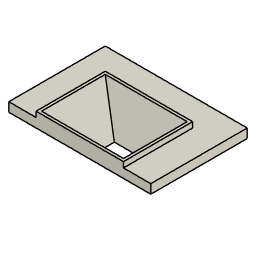
smarties_hopper (Autodesk Fusion 360 design; units mm, degrees)
part number: 2025-05-19-10-29-37-314
Autodesk Fusion 360 part; units mm, degrees
sketch "Bottom opening" plane through (0, 0, 0) normal (0, 0, 1) x (1, 0, 0)
  line L0 (0, 0) -> (25, 0)
  line L1 (25, 0) -> (25, 25)
  line L2 (25, 25) -> (0, 25)
  line L3 (0, 25) -> (0, 0)
  line L4 (-4, 29) -> (29, 29)
  line L5 (29, 29) -> (29, -4)
  line L6 (29, -4) -> (-4, -4)
  line L7 (-4, -4) -> (-4, 29)
  dimension "d3" = 25
  dimension "d4" = 25
  dimension "d5" = 4
  dimension "d6" = 4
  dimension "d7" = 4
  dimension "d8" = 4
  constraint horizontal L0
  constraint vertical L1
  constraint horizontal L2
  constraint vertical L3
  constraint coincident L0.start L3.end
  constraint horizontal L4
  constraint vertical L5
  constraint horizontal L6
  constraint vertical L7
  measures "d3" distance of L0.start L0.end
  measures "d4" distance of L0.end L1.end
  measures "d5" distance of L2 L4
  measures "d6" distance of L0 L6
  measures "d7" distance of L1 L5
  measures "d8" distance of L3 L7
ref_plane "WorkPlane1" through (0, 0, 37) normal (0, 0, 1) x (1, 0, 0)
sketch "Top opening" plane through (0, 0, 37) normal (0, 0, 1) x (1, 0, 0)
  line L0 (25, 25) -> (0, 25)
  line L1 (25, 0) -> (25, 25)
  line L2 (0, 0) -> (25, 0)
  line L3 (0, 25) -> (0, 0)
  line L4 (-4, 29) -> (29, 29)
  line L5 (29, -4) -> (-4, -4)
  line L6 (29, 29) -> (29, -4)
  line L7 (-4, -4) -> (-4, 29)
  line L8 (-32.5, 47.5) -> (57.5, 47.5)
  line L9 (57.5, 47.5) -> (57.5, -22.5)
  line L10 (57.5, -22.5) -> (-32.5, -22.5)
  line L11 (-32.5, -22.5) -> (-32.5, 47.5)
  line L12 (-35.5, 50.5) -> (60.5, 50.5)
  line L13 (60.5, 50.5) -> (60.5, -25.5)
  line L14 (60.5, -25.5) -> (-35.5, -25.5)
  line L15 (-35.5, -25.5) -> (-35.5, 50.5)
  line L16 (-36.5, 51.5) -> (61.5, 51.5)
  line L17 (61.5, 51.5) -> (61.5, -26.5)
  line L18 (61.5, -26.5) -> (-36.5, -26.5)
  line L19 (-36.5, -26.5) -> (-36.5, 51.5)
  dimension "d14" = 3
  dimension "d15" = 4
  dimension "d16" = 3
  dimension "d17" = 4
  dimension "d18" = 90
  dimension "d19" = 70
  dimension "d20" = 3
  dimension "d21" = 4
  dimension "d22" = 3
  dimension "d23" = 4
  dimension "d24" = 28.5
  dimension "d25" = 28.5
  dimension "d26" = 18.5
  dimension "d27" = 18.5
  constraint horizontal L8
  constraint vertical L9
  constraint horizontal L10
  constraint vertical L11
  constraint horizontal L12
  constraint vertical L13
  constraint horizontal L14
  constraint vertical L15
  constraint horizontal L16
  constraint vertical L17
  constraint horizontal L18
  constraint vertical L19
  measures "d14" distance of L9 L13
  measures "d15" distance of L9 L17
  measures "d16" distance of L11 L15
  measures "d17" distance of L11 L19
  measures "d18" distance of L8.start L8.end
  measures "d19" distance of L8.end L9.end
  measures "d20" distance of L8 L12
  measures "d21" distance of L8 L16
  measures "d22" distance of L10 L14
  measures "d23" distance of L10 L18
  measures "d24" distance of L7 L11
  measures "d25" distance of L6 L9
  measures "d26" distance of L4 L8
  measures "d27" distance of L5 L10
loft "Loft1" add profiles "Top opening", "Bottom opening" section 1 contours L8 L9 L10 L11 | L12 L13 L14 L15 | L16 L17 L18 L19 section 2 contours L0 L1 L2 L3 | L4 L5 L6 L7
extrude "Extrude1" cut sketch "Top opening" against normal blind 6 contours L16 L17 L18 L19
sketch "Support lip" plane through (60.5, 0, 0) normal (1, 0, 0) x (0, 1, 0)
  line L0 (-25.5, 35.8615) -> (50.5, 35.8615)
  line L1 (50.5, 35.8615) -> (50.5, 37)
  line L2 (50.5, 37) -> (-25.5, 37)
  line L3 (-25.5, 37) -> (-25.5, 35.8615)
  line L4 (-25.5, 31) -> (80.5, 31)
  line L5 (80.5, 31) -> (80.5, 21)
  line L6 (80.5, 21) -> (-25.5, 21)
  line L7 (-25.5, 21) -> (-25.5, 31)
  dimension "d31" = 6
  dimension "d34" = 10
  dimension "d35" = 30
  constraint horizontal L4
  constraint vertical L5
  constraint horizontal L6
  constraint vertical L7
  constraint collinear L3 L7
  measures "d31" distance of L2 L4
  measures "d34" distance of L4.start L6.end
  measures "d35" horizontal distance of L1.end L4.end
extrude "Extrude2" add sketch "Support lip" along normal blind 30 and the other way blind 126 contours L4 L5 L6 L7
loft "Loft2" cut profiles "Top opening", "Bottom opening" section 1 contours L8 L9 L10 L11 section 2 contours L0 L1 L2 L3
extrude "Extrude3" add 1 faces at (-2.5, 49.5, 37) along direction (0, 0, -1) blind 6
equation "bottom_outlet_size = 25 mm" comment "The side lengths of the bottom opening of the Smartie Hopper."
equation "hopper_wall_thickness = 4 mm" comment "The thickness of the hopper walls used for the \"loft\" function."
equation "d3 = bottom_outlet_size"
equation "d4 = bottom_outlet_size"
equation "d5 = hopper_wall_thickness"
equation "d6 = hopper_wall_thickness"
equation "d7 = hopper_wall_thickness"
equation "d8 = hopper_wall_thickness"
equation "hopper_height = 37 mm" comment "Distance between the top and bottom openings of the Smartie Hopper."
equation "d10 = hopper_height"
equation "acrylic_thickness = 3 mm" comment "Thickness of the clear acrylic panels used for the Unsorted Smarties Holder."
equation "top_outlet_width = 90 mm" comment "The width of the top opening of the Smartie Hopper."
equation "top_outlet_depth = 70 mm" comment "The depth of the top opening of the Smartie Hopper."
equation "d14 = acrylic_thickness"
equation "d15 = hopper_wall_thickness"
equation "d16 = acrylic_thickness"
equation "d17 = hopper_wall_thickness"
equation "d18 = top_outlet_width"
equation "d19 = top_outlet_depth"
equation "d20 = acrylic_thickness"
equation "d21 = hopper_wall_thickness"
equation "d22 = acrylic_thickness"
equation "d23 = hopper_wall_thickness"
equation "d24 = ( top_outlet_width - ( bottom_outlet_size + 2 * hopper_wall_thickness ) ) / 2"
equation "d26 = ( top_outlet_depth - ( bottom_outlet_size + 2 * hopper_wall_thickness ) ) / 2"
equation "MDF_thickness = 6 mm" comment "Thickness of the MDF panels used for the construction of the mini arcade game enclosure."
equation "d29 = -MDF_thickness"
equation "d31 = MDF_thickness"
equation "support_lip_width = 30 mm" comment "The depth that the suport lip should extend beneath the Colour Detection Mechanism Top Panel."
equation "support_lip_thickness = 10 mm" comment "The thickness of the support lip."
equation "d34 = support_lip_thickness"
equation "d35 = support_lip_width"
equation "d36 = support_lip_width"
equation "d38 = ( top_outlet_width + 2 * acrylic_thickness ) + support_lip_width"
equation "d40 = -MDF_thickness"
named bodies: "Smarties Hopper"
